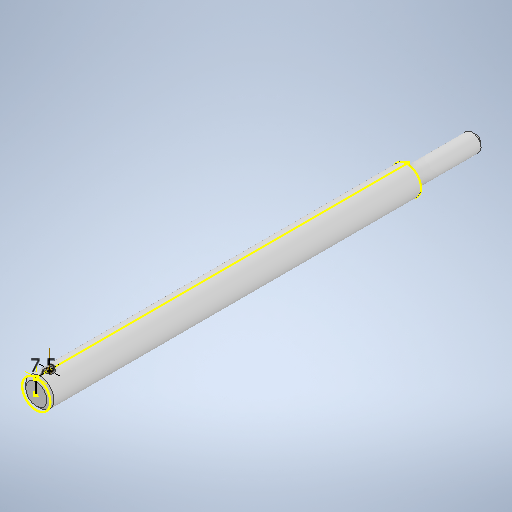
# Autodesk Inventor part: tłok
Saved by Autodesk Inventor 2025 (Build 290162000, 162)
## iProperties
Created: 2025-03-17
Part Number: tłok
Material: Ogólny
Document SubType Name: Modeling
Designer: marci
Density: 1 g/cm^3
Appearance: Domyślna
Author: marci
Autodesk Inventor part; units mm, degrees
ref_plane "YZ Plane" through (0, 0, 0) normal (1, 0, 0) x (0, 1, 0)
ref_plane "XZ Plane" through (0, 0, 0) normal (0, 1, 0) x (-1, 0, 0)
ref_plane "XY Plane" through (0, 0, 0) normal (0, 0, 1) x (1, 0, 0)
sketch "Szkic1" plane through (0, 0, 0) normal (0, 0, 1) x (1, 0, 0)
  circle A0 centre (0, 0) radius 8
  dimension "d0" = 16
  constraints: 1 centre point, 1 coincident
  measures "d0" diameter of A0
extrude "Wyciągnięcie proste1" add sketch "Szkic1" against normal blind 210
sketch "Szkic2" plane through (0, 0, 0) normal (0, 0, 1) x (1, 0, 0)
  line L0 (0, 0) -> (0, 8)
  circle A0 centre (0, 0) radius 8 projected
  circle A1 centre (0, 0) radius 8 projected
  circle A2 centre (0, 0) radius 8 projected
  constraints: 2 end point, 1 vertical, 1 vertical alignment, 1 other
sketch3d "Szkic 3D1"
sketch3d "Szkic 3D2"
sketch "Szkic4" plane through (0, 0, 0) normal (0, 0, 1) x (1, 0, 0)
  circle A0 centre (0, 0) radius 8 projected
  circle A1 centre (0, 0) radius 8 projected
  point P0 (0, 8)
hole "Otwór1" at (0, 8, -7.5) direction (0, -1, 0) diameter 5 end through all
chamfer "Faza2" distance 2 angle 45 1 edges at (-8, 0, 0)
sketch "Szkic6" plane through (0, 0, -210) normal (0, 0, -1) x (-1, 0, 0)
  point P0 (0, 0)
sketch "Szkic9" plane through (0, 0, -210) normal (0, 0, -1) x (-1, 0, 0)
  circle A0 centre (0, 0) radius 5
  dimension "d27" = 10
  constraints: 1 centre point, 1 coincident
  measures "d27" diameter of A0
extrude "Wyciągnięcie proste4" add sketch "Szkic9" along normal blind 37
sketch "Szkic10" plane through (0, 0, -247) normal (0, 0, -1) x (-1, 0, 0)
  circle A0 centre (0, 0) radius 3
  dimension "d30" = 6
  constraints: 1 centre point, 1 coincident
  measures "d30" diameter of A0
extrude "Wyciągnięcie proste5" add sketch "Szkic10" along normal blind 2
draft "Pochylenie ściany1" angle 45 pull direction (0, 0, -1) faces at (-2.9903, -0.2414, -248.3333) fixed edges at (3, 0, -249)
